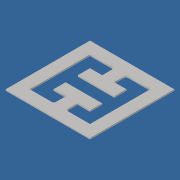
# Autodesk Inventor part: Logo Inlay
Saved by Autodesk Inventor 2016 (Build 200138000, 138)
## iProperties
Created: 2015-10-27
Part Number: Logo Inlay
Material: Generic
Document SubType Name: Modeling
Designer: Sam Clay
Density: 1 g/cm^3
Appearance: Default
Author: Sam Clay
Autodesk Inventor part; units mm, degrees
ref_plane "YZ Plane" through (0, 0, 0) normal (1, 0, 0) x (0, 1, 0)
ref_plane "XZ Plane" through (0, 0, 0) normal (0, 1, 0) x (-1, 0, 0)
ref_plane "XY Plane" through (0, 0, 0) normal (0, 0, 1) x (1, 0, 0)
sketch "Sketch1" plane through (0, 0, 0) normal (0, 1, 0) x (-1, 0, 0)
  line L0 (0.0001, 0.003) -> (0.0001, 0)
  line L1 (0.0001, -17.064) -> (-0.002, -0.0021)
  line L2 (-2.3966, -2.4008) -> (-2.3966, -14.6631)
  line L3 (-2.3966, -14.6631) -> (-6.8866, -14.6631)
  spline S0 degree 3 poles (-6.8866, -14.6631) (-7.1334, -14.6502) (-7.3283, -14.4466) (-7.3261, -14.1977) knots 2 2 2 2 3 3 3 3
  line L4 (-6.8866, -14.6631) -> (-7.1334, -14.6502) construction
  line L5 (-7.1334, -14.6502) -> (-7.3283, -14.4466) construction
  line L6 (-7.3283, -14.4466) -> (-7.3261, -14.1977) construction
  line L7 (-7.2677, -7.2678) -> (-4.8517, -7.2677)
  line L8 (-9.7961, -9.7964) -> (-12.2057, -9.7985)
  line L9 (-4.8515, -9.7963) -> (-9.7961, -9.7964)
  line L10 (-4.8515, -12.2081) -> (-4.8515, -9.7963)
  line L11 (-7.3261, -12.2103) -> (-4.8515, -12.2081)
  line L12 (-7.3261, -14.1977) -> (-7.3261, -12.2103)
  line L13 (-12.2057, -9.7985) -> (-12.206, -12.2102)
  line L14 (-17.0619, -17.062) -> (0.0001, -17.064)
  line L15 (-12.206, -12.2102) -> (-9.7379, -12.2102)
  line L16 (-9.7379, -12.2102) -> (-9.7379, -14.228)
  line L17 (-9.7379, -14.228) -> (-9.7509, -14.4705) construction
  spline S1 degree 3 poles (-9.7379, -14.228) (-9.7509, -14.4705) (-9.9544, -14.661) (-10.2034, -14.6631) knots 11 11 11 11 12 12 12 12
  line L18 (-9.7509, -14.4705) -> (-9.9544, -14.661) construction
  line L19 (-9.9544, -14.661) -> (-10.2034, -14.6631) construction
  line L20 (-14.6632, -14.6631) -> (-14.6675, -14.6631)
  line L21 (-10.2034, -14.6631) -> (-14.6632, -14.6631)
  line L22 (-17.064, 0.0001) -> (-17.0619, -17.062)
  line L23 (-12.206, -7.2698) -> (-7.2677, -7.2678)
  line L24 (-14.6675, -14.6631) -> (-14.6676, -2.4008)
  line L25 (-12.206, -4.8538) -> (-12.206, -7.2698)
  line L26 (-9.7357, -2.8642) -> (-9.738, -4.8538)
  line L27 (-9.738, -4.8538) -> (-12.206, -4.8538)
  line L28 (-9.7357, -2.6174) -> (-9.7357, -2.8642) construction
  spline S2 degree 3 poles (-10.1731, -2.4009) (-9.9285, -2.4159) (-9.7357, -2.6174) (-9.7357, -2.8642) knots 16 16 16 16 17 17 17 17
  line L29 (-10.1731, -2.4009) -> (-9.9285, -2.4159) construction
  line L30 (-9.9285, -2.4159) -> (-9.7357, -2.6174) construction
  line L31 (-14.6676, -2.4008) -> (-10.1731, -2.4009)
  line L32 (-0.002, -0.0021) -> (0.0001, 0)
  line L33 (0.0001, 0) -> (-17.064, 0.0001)
  line L34 (-4.8517, -7.2677) -> (-4.8516, -4.8558)
  line L35 (-7.3282, -4.8559) -> (-7.3282, -2.8294)
  line L36 (-4.8536, -4.8537) -> (-7.3282, -4.8559)
  line L37 (-7.3087, -2.5977) -> (-7.1248, -2.4138) construction
  spline S3 degree 3 poles (-7.3282, -2.8294) (-7.3087, -2.5977) (-7.1248, -2.4138) (-6.893, -2.3986) knots 26 26 26 26 27 27 27 27
  line L38 (-7.3282, -2.8294) -> (-7.3087, -2.5977) construction
  line L39 (-7.1248, -2.4138) -> (-6.893, -2.3986) construction
  line L40 (-4.8516, -4.8558) -> (-4.8536, -4.8537)
  line L41 (-6.893, -2.3986) -> (-2.3985, -2.3986)
  line L42 (-2.3985, -2.3986) -> (-2.3964, -2.4007)
  line L43 (-2.3964, -2.4007) -> (-2.3966, -2.4008)
  line L44 (15.402, -0.0001) -> (-1.6922, 0)
  dimension "d2" = 17.0942
  constraints: 66 end point, 13 other
  measures "d2" distance of L44.start L44.end
extrude "Extrusion1" add sketch "Sketch1" along normal blind 0.254
body "Solid1"
